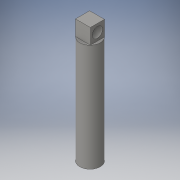
# Autodesk Inventor part: cylendar
Saved by Autodesk Inventor 2016 (Build 200138000, 138)
## iProperties
Created: 2018-01-10
Part Number: cylendar
Material: Aluminum 6061
Document SubType Name: Modeling
Designer: New User
Density: 2.7 g/cm^3
Appearance: Aluminum - Flat
Mass: 1336.57 g
Surface Area: 699.702 cm^2
Volume: 495.027 cm^3
Author: New User
Autodesk Inventor part; units mm, degrees
ref_plane "YZ Plane" through (0, 0, 0) normal (1, 0, 0) x (0, 1, 0)
ref_plane "XZ Plane" through (0, 0, 0) normal (0, 1, 0) x (-1, 0, 0)
ref_plane "XY Plane" through (0, 0, 0) normal (0, 0, 1) x (1, 0, 0)
sketch "Sketch1" plane through (0, 0, 0) normal (0, 1, 0) x (-1, 0, 0)
  circle A0 centre (0, 0) radius 25.4
  dimension "d0" = 50.8
  constraints: 1 centre point, 1 coincident
  measures "d0" diameter of A0
extrude "Extrusion1" add sketch "Sketch1" along normal blind 266.7
sketch "Sketch2" plane through (0, 266.7, 0) normal (0, 1, 0) x (1, 0, 0)
  circle A0 centre (0, 0) radius 25.4 projected
  line L0 (-18.3739, -17.5374) -> (18.3739, -17.5374)
  line L1 (18.3739, -17.5374) -> (18.3739, 17.5374)
  line L2 (18.3739, 17.5374) -> (-18.3739, 17.5374)
  line L3 (-18.3739, 17.5374) -> (-18.3739, -17.5374)
  line L4 (-18.3739, -17.5374) -> (18.3739, 17.5374) construction
  line L5 (18.3739, -17.5374) -> (-18.3739, 17.5374) construction
  constraints: 12 end point, 2 midpoint, 2 parallel, 1 horizontal, 1 perpendicular, 2 other
extrude "Extrusion4" add sketch "Sketch2" along normal blind 38.1 contours L1 L0 L3 L2
sketch "Sketch4" plane through (18.3739, 266.7, 17.5374) normal (1, 0, 0) x (0, 0, -1)
  circle A0 centre (17.5374, 19.05) radius 12.7
  point P0 (17.5374, -266.7)
  dimension "d10" = 25.4
  constraints: 1 centre point
  measures "d10" diameter of A0
extrude "Extrusion5" cut sketch "Sketch4" against normal blind 38.1
sketch "Sketch5" plane through (0, 0, 0) normal (0, -1, 0) x (1, 0, 0)
  circle A0 centre (0, 0) radius 9.525
  dimension "d13" = 19.05
  constraints: 1 centre point, 1 coincident
  measures "d13" diameter of A0
extrude "Extrusion6" cut sketch "Sketch5" against normal blind 266.7
body "Solid1"
